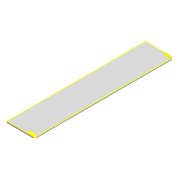
# Autodesk Inventor part: Bending_plate
Saved by Autodesk Inventor 2022 (Build 260153000, 153)
## iProperties
Created: 2022-07-29
Part Number: Bending_plate
Material: Generic
Document SubType Name: Modeling
Designer: dell
Density: 1 g/cm^3
Appearance: Default
Author: dell
Autodesk Inventor part; units mm, degrees
ref_plane "YZ Plane" through (0, 0, 0) normal (1, 0, 0) x (0, 1, 0)
ref_plane "XZ Plane" through (0, 0, 0) normal (0, 1, 0) x (-1, 0, 0)
sketch "Sketch1" plane through (0, 0, 0) normal (0, 1, 0) x (-1, 0, 0)
  line L0 (0, 0) -> (100, 0)
  line L1 (100, 0) -> (100, -500)
  line L2 (100, -500) -> (0, -500)
  line L3 (0, -500) -> (0, 0)
  dimension "d0" = 500
  dimension "d1" = 100
  constraints: 8 end point, 2 parallel, 1 horizontal, 1 perpendicular
  measures "d0" distance of L2.end L0.start
  measures "d1" distance of L1.end L2.end
extrude "Extrusion1" add sketch "Sketch1" along normal blind 6
sketch "Sketch2" plane through (0, 6, 0) normal (0, 1, 0) x (1, 0, 0)
  circle A0 centre (-10, 5) radius 1.475
  line L0 (-100, 0) -> (0, 0) projected
  line L1 (0, 0) -> (0, 500) projected
  dimension "d4" = 2.95
  dimension "d5" = 5
  dimension "d6" = 10
  constraints: 1 centre point
  measures "d4" diameter of A0
  measures "d5" distance from line of L0 A0.centre
  measures "d6" distance from line of L1 A0.centre
extrude "Extrusion2" cut sketch "Sketch2" against normal blind 10
pattern_linear "Rectangular Pattern1" count 3 spacing 6 along (-1, 0, 0) of "Extrusion2"
ref_plane "Work Plane1" through (-100, 0, -250) normal (0, 0, 1) x (1, 0, 0)
sketch "Sketch3" plane through (0, 6, 0) normal (0, 1, 0) x (1, 0, 0)
  line L0 (-100, 0) -> (0, 0) projected
  line L1 (0, 0) -> (-4, 0)
  line L2 (-4, 0) -> (-4, 5)
  line L3 (-4, 5) -> (0, 5)
  line L4 (0, 5) -> (0, 0)
  dimension "d12" = 4
  dimension "d13" = 5
  constraints: 8 end point, 2 parallel, 1 horizontal, 1 perpendicular
  measures "d12" distance between parallel lines of L4 L2
  measures "d13" distance between parallel lines of L0 L3
extrude "Extrusion3" cut sketch "Sketch3" against normal blind 100
mirror "Mirror1" about plane through (-100, 0, -250) normal (0, 0, 1) of "Extrusion2", "Rectangular Pattern1", "Extrusion3"
sketch "Sketch4" plane through (0, 6, 0) normal (0, 1, 0) x (1, 0, 0)
  circle A0 centre (-22, 5) radius 1.475 projected
  circle A1 centre (-16, 5) radius 1.475 projected
  circle A2 centre (-10, 5) radius 1.475 projected
  line L0 (0, 495) -> (-4, 495) projected
  line L1 (-4, 495) -> (-4, 500) projected
  line L2 (-4, 500) -> (-100, 500) projected
  line L3 (-100, 500) -> (-100, 0) projected
  line L4 (-100, 0) -> (-4, 0) projected
  line L5 (-4, 0) -> (-4, 5) projected
  line L6 (-4, 5) -> (0, 5) projected
  line L7 (0, 5) -> (0, 495) projected
  circle A3 centre (-10, 495) radius 1.475 projected
  circle A4 centre (-16, 495) radius 1.475 projected
  circle A5 centre (-22, 495) radius 1.475 projected
  point P0 (0, 0)
body "Solid1"
